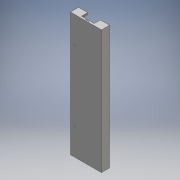
# Autodesk Inventor part: Base
Saved by Autodesk Inventor 2016 (Build 200138000, 138)
## iProperties
Created: 2015-08-31
Part Number: Base
Material: Generic
Document SubType Name: Modeling
Designer: amatiasq
Density: 1 g/cm^3
Appearance: Default
Author: amatiasq
Autodesk Inventor part; units mm, degrees
ref_plane "YZ Plane" through (0, 0, 0) normal (1, 0, 0) x (0, 1, 0)
ref_plane "XZ Plane" through (0, 0, 0) normal (0, 1, 0) x (-1, 0, 0)
ref_plane "XY Plane" through (0, 0, 0) normal (0, 0, 1) x (1, 0, 0)
sketch "Sketch1" plane through (0, 0, 0) normal (0, 1, 0) x (-1, 0, 0)
  line L0 (0, 0) -> (-50, 0)
  line L1 (-50, 0) -> (-50, -200)
  line L2 (-50, -200) -> (0, -200)
  line L3 (0, -200) -> (0, 0)
  dimension "d0" = 50
  dimension "d1" = 200
  constraints: 8 end point, 2 parallel, 1 horizontal, 1 perpendicular
  measures "d0" distance of L2.end L1.end
  measures "d1" distance of L1.end L0.end
extrude "Base" add sketch "Sketch1" along normal blind 3
sketch "Sketch4" plane through (0, 3, 0) normal (0, 1, 0) x (1, 0, 0)
  line L0 (0, 0) -> (50, 0) projected
  line L1 (50, 0) -> (50, 200) projected
  line L2 (50, 200) -> (0, 200) projected
  line L3 (0, 200) -> (0, 0) projected
  line L4 (3, 3) -> (47, 3)
  line L5 (47, 3) -> (47, 197)
  line L6 (47, 197) -> (3, 197)
  line L7 (3, 197) -> (3, 3)
  line L8 (14.7, 0) -> (35.3, 0)
  line L9 (35.3, 0) -> (35.3, 3)
  line L10 (35.3, 3) -> (14.7, 3)
  line L11 (14.7, 3) -> (14.7, 0)
  point P0 (25, 0)
  point P1 (25, 3)
  dimension "d6" = 3
  dimension "d7" = 20.6
  constraints: 16 end point, 4 midpoint, 2 parallel, 1 horizontal, 1 perpendicular, 3 other
  measures "d6" distance between parallel lines of L3 L7
  measures "d7" distance between parallel lines of L9 L11
extrude "Paredes" add sketch "Sketch4" along normal blind 10 contours L3 L2 L1 L0 L9 L4 L5 L6 L7 L11
sketch "Sketch5" plane through (0, 3, 0) normal (0, 1, 0) x (1, 0, 0)
  line L0 (22.5, 0) -> (27.5, 0)
  line L1 (27.5, 0) -> (27.5, 197)
  line L2 (27.5, 197) -> (22.5, 197)
  line L3 (22.5, 197) -> (22.5, 0)
  line L4 (14.7, 0) -> (35.3, 0) projected
  line L5 (47, 197) -> (3, 197) projected
  point P0 (0, 0)
  point P1 (25, 0)
  point P2 (25, 197)
  dimension "d10" = 5
  constraints: 8 end point, 4 midpoint, 2 parallel, 1 horizontal, 1 perpendicular
  measures "d10" distance between parallel lines of L1 L3
extrude "Canal" cut sketch "Sketch5" against normal blind 1.5
sketch "Sketch6" plane through (0, 3, 0) normal (0, 1, 0) x (1, 0, 0)
  line L0 (7, 3.0083) -> (7, 197)
  line L1 (22.5, 197) -> (3, 197) projected
  line L2 (3, 197) -> (3, 3) projected
  line L3 (3, 3) -> (14.7, 3) projected
  point P0 (0, 0)
  point P1 (7, 43)
  point P2 (7, 157)
  dimension "d13" = 4
  dimension "d14" = 40
  dimension "d15" = 40
  constraints: 3 point on line, 2 end point, 1 vertical
  measures "d13" distance between parallel lines of L0 L2
  measures "d14" distance from line of L3 point (7, 43)
  measures "d15" distance from line of L1 point (7, 157)
hole "Agujeros" at (7, 3, -43) at (7, 3, -157) direction (0, -1, 0) diameter 2 end through all
equation "\"d0\" = base_ancho"
equation "\"d1\" = base_largo"
equation "\"d2\" = base_alto"
equation "\"d6\" = muros_grosor"
equation "\"d7\" = hoja_ancho + 2 * margen"
equation "\"d8\" = muros_alto"
equation "\"d10\" = rail_grosor"
equation "\"d11\" = rail_alto"
equation "\"d21\" = d14"
equation "\"margen\" = 0.3"
equation "\"hoja_stop_largo\" = 5"
equation "\"hoja_stop_saliente\" = 5"
equation "\"hoja_stop_posicion\" = 5"
equation "\"hoja_alto\" = 3"
equation "\"rail_grosor\" = 5"
equation "\"base_alto\" = 3"
equation "\"base_ancho\" = 50"
equation "\"base_largo\" = 200"
equation "\"muros_alto\" = 10"
equation "\"muros_grosor\" = 3"
equation "\"rail_alto\" = 1.5"
equation "\"hoja_stop_biselado\" = 2"
equation "\"hoja_cola_biselado\" = 1"
equation "\"hoja_filo_biselado\" = 0.5"
equation "\"hoja_ancho\" = 20"
body "Solid1"
